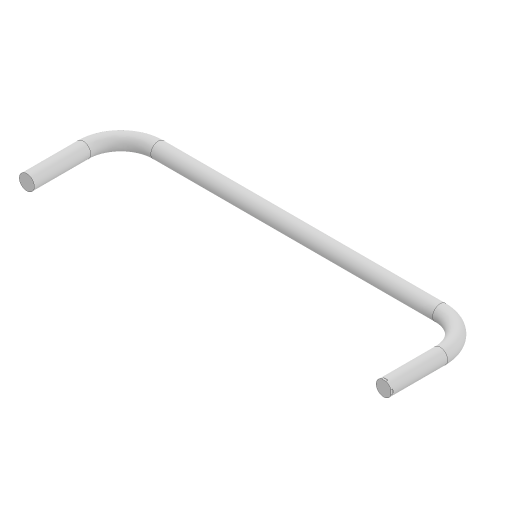
# Autodesk Inventor part: Handle
Saved by Autodesk Inventor 2024.3 (Build 283343000, 343)
## iProperties
Created: 2025-10-02
Part Number: Handle
Material: Generic
Document SubType Name: Modeling
Designer: ajclo
Density: 1 g/cm^3
Appearance: Default
Author: ajclo
Autodesk Inventor part; units mm, degrees
ref_plane "YZ Plane" through (0, 0, 0) normal (1, 0, 0) x (0, 1, 0)
ref_plane "XZ Plane" through (0, 0, 0) normal (0, 1, 0) x (-1, 0, 0)
ref_plane "XY Plane" through (0, 0, 0) normal (0, 0, 1) x (1, 0, 0)
sketch "Sketch1" plane through (0, 0, 0) normal (1, 0, 0) x (0, 1, 0)
  circle A0 centre (0, 0) radius 4
  dimension "d0" = 8
  constraints: 1 centre point, 1 coincident
  measures "d0" diameter of A0
extrude "Extrusion1" add sketch "Sketch1" along normal mid plane 150
sketch "Sketch4" plane through (75, 0, 0) normal (1, 0, 0) x (0, 0, -1)
  circle A0 centre (0, 0) radius 4
  line L0 (-20, 15.4363) -> (-20, -7.2727)
  circle A1 centre (0, 0) radius 4 projected
  dimension "d10" = 20
  dimension "d11" = 0
  constraints: 2 end point, 1 centre point, 1 coincident, 1 vertical
  measures "d10" distance from line of point (0, 0) L0
  measures "d11" radial gap between concentric circles of A1 A0
revolve "Revolution1" add sketch "Sketch4" angle 90 about axis through (75, 15.4363, 20) along (0, -1, 0)
mirror "Mirror1" about plane through (0, 0, 0) normal (1, 0, 0) of "Revolution1"
sketch "Sketch5" plane through (95, 0, 20) normal (0, 0, 1) x (1, 0, 0)
  circle A0 centre (0, 0) radius 4 projected
  point P0 (-95, 0)
extrude "Extrusion3" add sketch "Sketch5" along normal blind 30
mirror "Mirror2" about plane through (0, 0, 0) normal (1, 0, 0) of "Extrusion3"
sketch "Sketch6" plane through (95, 0, 50) normal (0, 0, 1) x (1, 0, 0)
  circle A0 centre (0, 0) radius 4 projected
  line L0 (-1.147, 3.832) -> (3.8236, 3.832)
  line L1 (3.8236, 3.832) -> (3.8236, -1.1749)
  line L2 (3.8236, -1.1749) -> (-1.147, -1.1749)
  line L3 (-1.147, -1.1749) -> (-1.147, 3.832)
  circle A1 centre (0, 0) radius 4 projected
  point P0 (-95, 0)
  point P1 (3.8236, 1.1749)
  point P2 (1.147, 3.832)
  constraints: 8 end point, 2 parallel, 2 point on circle, 1 horizontal, 1 perpendicular
extrude "Extrusion4" cut sketch "Sketch6" against normal blind 1 contours A0 L0 | L1 A0
body "Solid1"
